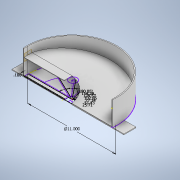
# Autodesk Inventor part: FlatRotationalTransferOldV
Saved by Autodesk Inventor 2020 (Build 240168000, 168)
## iProperties
Created: 2021-03-21
Part Number: FlatRotationalTransferOldV
Material: Generic
Document SubType Name: Sheet Metal
Designer: tdmp4
Density: 1 g/cm^3
Appearance: Default
Sheet Metal Rule: Default
Author: tdmp4
Autodesk Inventor part; units mm, degrees
ref_plane "YZ Plane" through (0, 0, 0) normal (1, 0, 0) x (0, 1, 0)
ref_plane "XZ Plane" through (0, 0, 0) normal (0, 1, 0) x (-1, 0, 0)
ref_plane "XY Plane" through (0, 0, 0) normal (0, 0, 1) x (1, 0, 0)
sketch "Sketch3" plane through (0, 0, 0) normal (0, 1, 0) x (-1, 0, 0)
  arc A0 (127.5964, -8.854) -> (151.8036, -8.854) centre (139.7, -12.7) ccw
  arc A1 (0, -12.7) -> (279.4, -12.7) centre (139.7, -12.7) ccw
  line L0 (279.4, -12.7) -> (279.4, 0)
  line L1 (279.4, 0) -> (151.8036, 0)
  line L2 (151.8036, 0) -> (151.8036, -8.854)
  line L3 (127.5964, 0) -> (0, 0)
  line L4 (0, 0) -> (0, -12.7)
  line L5 (127.5964, 0) -> (127.5964, -8.854)
  point P0 (0, -12.7)
  dimension "d9" = 279.4
  constraints: 12 end point, 4 point on circle, 3 vertical, 2 centre point, 2 perpendicular, 1 coincident, 1 point on line
  measures "d9" diameter of A1
extrude "Extrusion2" add sketch "Sketch3" along normal blind 2.54
sketch "Sketch4" plane through (0, 2.54, 0) normal (0, 1, 0) x (1, 0, 0)
  arc A0 (-127.5964, 8.854) -> (-151.8036, 8.854) centre (-139.7, 12.7) ccw projected
  arc A1 (0, 12.7) -> (-279.4, 12.7) centre (-139.7, 12.7) ccw
  line L0 (-127.5964, 0) -> (0, 0) projected
  line L1 (0, 0) -> (2.54, 0)
  line L2 (-279.4, 12.7) -> (-279.4, 0) projected
  line L3 (-279.4, 0) -> (-281.94, 0)
  circle A2 centre (-139.7, 12.7) radius 142.8058
  line L4 (0, 0) -> (2.54, 0)
  line L5 (0, 0) -> (0, 12.7)
  arc A3 (0, 12.7) -> (-279.4, 12.7) centre (-139.7, 12.7) ccw projected
  line L6 (-279.4, 0) -> (-279.4, 12.7)
  line L7 (-279.4, 0) -> (-281.94, 0)
  dimension "d12" = 2.54
  dimension "d13" = 2.54
  constraints: 13 end point, 3 point on circle, 2 coincident, 2 collinear, 2 point on line, 1 centre point, 1 horizontal, 1 perpendicular, 1 vertical, 3 other
  measures "d12" distance of L0.end L1.end
  measures "d13" distance of L2.end L3.end
extrude "Extrusion3" add sketch "Sketch4" along normal blind 76.2 contours A1 L2 L3 A2 L1 L5 picked at (-280.1039, 19.3593)
sketch "Sketch6" plane through (-279.4, 0, -12.7) normal (-1, 0, 0) x (0, 0, 1)
  line L0 (12.7, 0) -> (3.846, 0) projected
  line L1 (0, 2.54) -> (-139.7, 2.54) projected
  line L2 (12.7, 0) -> (-25.4, 0)
  line L3 (-25.4, 0) -> (-25.4, 2.54)
  line L4 (-25.4, 2.54) -> (12.7, 2.54)
  line L5 (12.7, 2.54) -> (12.7, 0)
  dimension "d16" = 38.1
  constraints: 8 end point, 2 parallel, 1 horizontal, 1 perpendicular, 1 point on line
  measures "d16" distance of L3.end L4.end
extrude "Extrusion4" add sketch "Sketch6" along normal mid plane 76.2
sketch "Sketch7" plane through (0, 0, 0) normal (1, 0, 0) x (0, 0, -1)
  line L0 (38.1, 0) -> (0, 0) projected
  line L1 (0, 0) -> (38.1, 0)
  line L2 (38.1, 0) -> (38.1, 2.54)
  line L3 (38.1, 2.54) -> (0, 2.54)
  line L4 (0, 2.54) -> (0, 0)
  dimension "d19" = 38.1
  dimension "d20" = 2.54
  constraints: 8 end point, 2 parallel, 1 horizontal, 1 perpendicular
  measures "d19" distance of L3.end L2.end
  measures "d20" distance of L1.end L2.end
extrude "Extrusion5" add sketch "Sketch7" along normal mid plane 76.2
sketch "Sketch8" plane through (0, 2.54, 0) normal (0, 1, 0) x (1, 0, 0)
  line L0 (-151.8036, 0) -> (-151.8036, 8.854) projected
  line L1 (-279.4, 0) -> (-151.8036, 0) projected
  line L2 (-151.8036, 0) -> (-279.4, 0)
  line L3 (-279.4, 0) -> (-279.4, 2.54)
  line L4 (-279.4, 12.7) -> (-279.4, 0) projected
  line L5 (-279.4, 2.54) -> (-151.8036, 2.54)
  line L6 (-151.8036, 2.54) -> (-151.8036, 0)
  arc A0 (-127.5964, 8.854) -> (-151.8036, 8.854) centre (-139.7, 12.7) ccw projected
  line L7 (-139.7, 12.7) -> (-15.4667, 72.5276)
  line L8 (-139.7, 12.7) -> (-1.8115, 12.7) construction
  line L9 (-139.7, 12.7) -> (-52.5985, 121.9219)
  arc A1 (-2.3285, 38.1) -> (-277.0715, 38.1) centre (-139.7, 12.7) ccw projected
  line L10 (-139.7, 12.7) -> (0, 12.7) construction
  line L11 (-139.7, 12.7) -> (-108.6138, 148.8974)
  line L12 (-139.7, 12.7) -> (0, 12.7) construction
  line L13 (-139.7, 12.7) -> (-170.7862, 148.8974)
  line L14 (-139.7, 12.7) -> (0, 12.7) construction
  line L15 (-139.7, 12.7) -> (-226.8015, 121.9219)
  line L16 (-139.7, 12.7) -> (0, 12.7) construction
  line L17 (-139.7, 12.7) -> (-265.5654, 73.3136)
  line L18 (-139.7, 12.7) -> (0, 12.7) construction
  line L19 (-139.7, 12.7) -> (-279.4, 12.7)
  line L20 (-139.7, 12.7) -> (0, 12.7) construction
  line L21 (-134.1897, 24.1423) -> (-105.865, 148.2407)
  line L22 (-127.3184, 15.526) -> (-11.7903, 68.8712)
  line L23 (-15.4667, 72.5276) -> (-11.0364, 74.6611)
  arc A2 (0.8288, 38.1) -> (-280.2288, 38.1) centre (-139.7, 12.7) ccw projected
  line L24 (-129.5192, 20.2922) -> (-47.6995, 121.9219)
  line L25 (-145.2103, 24.1423) -> (-173.535, 148.2407)
  line L26 (-149.8808, 20.2922) -> (-231.2375, 122.3102)
  line L27 (-152.0816, 15.526) -> (-266.5148, 71.3012)
  line L28 (-152.0816, 15.526) -> (-282.4779, 15.526)
  arc A3 (2.54, 0) -> (-281.94, 0) centre (-139.7, 12.7) ccw projected
  line L29 (-151.8036, 0) -> (-151.8036, 8.854)
  line L30 (-279.4, 0) -> (-151.8036, 0)
  line L31 (-151.8036, 0) -> (-279.4, 0)
  line L32 (-279.4, 0) -> (-279.4, 2.54)
  line L33 (-279.4, 12.7) -> (-279.4, 0)
  line L34 (-279.4, 2.54) -> (-151.8036, 2.54)
  line L35 (-151.8036, 2.54) -> (-151.8036, 0)
  arc A4 (-127.5964, 8.854) -> (-151.8036, 8.854) centre (-139.7, 12.7) ccw
  line L36 (-139.7, 12.7) -> (-15.4667, 72.5276)
  line L37 (-139.7, 12.7) -> (-1.8115, 12.7) construction
  line L38 (-139.7, 12.7) -> (-52.5985, 121.9219)
  arc A5 (-2.3285, 38.1) -> (-277.0715, 38.1) centre (-139.7, 12.7) ccw
  line L39 (-139.7, 12.7) -> (0, 12.7) construction
  line L40 (-139.7, 12.7) -> (-108.6138, 148.8974)
  line L41 (-139.7, 12.7) -> (0, 12.7) construction
  line L42 (-139.7, 12.7) -> (-170.7862, 148.8974)
  line L43 (-139.7, 12.7) -> (0, 12.7) construction
  line L44 (-139.7, 12.7) -> (-226.8015, 121.9219)
  line L45 (-139.7, 12.7) -> (0, 12.7) construction
  line L46 (-139.7, 12.7) -> (-265.5654, 73.3136)
  line L47 (-139.7, 12.7) -> (0, 12.7) construction
  line L48 (-139.7, 12.7) -> (-279.4, 12.7)
  line L49 (-139.7, 12.7) -> (0, 12.7) construction
  line L50 (-134.1897, 24.1423) -> (-105.865, 148.2407)
  line L51 (-127.3184, 15.526) -> (-11.7903, 68.8712)
  line L52 (-15.4667, 72.5276) -> (-11.0364, 74.6611)
  arc A6 (0.8288, 38.1) -> (-280.2288, 38.1) centre (-139.7, 12.7) ccw
  line L53 (-129.5192, 20.2922) -> (-47.6995, 121.9219)
  line L54 (-145.2103, 24.1423) -> (-173.535, 148.2407)
  line L55 (-149.8808, 20.2922) -> (-231.2375, 122.3102)
  line L56 (-152.0816, 15.526) -> (-266.5148, 71.3012)
  line L57 (-152.0816, 15.526) -> (-282.4779, 15.526)
  arc A7 (2.54, 0) -> (-281.94, 0) centre (-139.7, 12.7) ccw
  arc A8 (-277.0715, 38.1) -> (-279.4, 12.7) centre (-139.7, 12.7) ccw projected
  line L58 (-279.4, 12.7) -> (-279.3714, 15.526)
  point P0 (0, 0)
  point P1 (-13.8346, 73.3136)
  point P2 (-128.2577, 18.2103)
  point P3 (0, 0)
  point P4 (-13.8346, 73.3136)
  point P5 (-128.2577, 18.2103)
  point P6 (-49.6477, 119.502)
  point P7 (-131.7817, 22.6293)
  point P8 (-136.874, 25.0816)
  point P9 (-142.526, 25.0816)
  point P10 (-229.3005, 119.8813)
  point P11 (-147.6183, 22.6293)
  point P12 (-151.1423, 18.2103)
  dimension "d23" = 2.54
  dimension "d24" = 25.714
  dimension "d25" = 51.429
  dimension "d26" = 77.143
  dimension "d27" = 102.857
  dimension "d28" = 128.571
  dimension "d29" = 154.286
  dimension "d30" = 180
  dimension "d33" = 2.54
  dimension "d34" = 25.714
  dimension "d35" = 51.429
  dimension "d36" = 77.143
  dimension "d37" = 102.857
  dimension "d38" = 128.571
  dimension "d39" = 154.286
  dimension "d40" = 180
  constraints: 112 end point, 27 point on circle, 20 horizontal, 14 equal length, 4 parallel, 4 perpendicular, 3 centre point, 3 point on line, 23 other
  measures "d23" distance of L1.start L3.end
  measures "d24" angle of L8 L7
  measures "d25" angle of L10 L9
  measures "d26" angle of L12 L11
  measures "d27" angle of L14 L13
  measures "d28" angle of L16 L15
  measures "d29" angle of L18 L17
  measures "d30" angle of L19 L20
  measures "d33" distance of L30.start L32.end
  measures "d34" angle of L37 L36
  measures "d35" angle of L39 L38
  measures "d36" angle of L41 L40
  measures "d37" angle of L43 L42
  measures "d38" angle of L45 L44
  measures "d39" angle of L47 L46
  measures "d40" angle of L48 L49
sketch "Sketch10" plane through (0, 2.54, 0) normal (0, 1, 0) x (1, 0, 0)
  arc A0 (-36.5718, 0) -> (-230.6482, 12.6651) centre (-133.61, 6.3326) ccw
  line L0 (-127.5964, 8.854) -> (-127.5964, 0) projected
  point P0 (0, 0)
  constraints: 2 point on circle, 1 centre point
sketch "Sketch11" plane through (0, 2.54, 0) normal (0, 1, 0) x (1, 0, 0)
  line L0 (-127.5964, 8.854) -> (-127.5964, 0) projected
  line L1 (-127.5964, 0) -> (-151.8036, 0)
  line L2 (-139.7, 12.7038) -> (-139.7, 0)
  point P0 (0, 0)
  constraints: 4 end point, 1 horizontal, 1 midpoint
sketch "Sketch9" plane through (-127.5964, 2.54, 0) normal (0, 0, 1) x (1, 0, 0)
  line L0 (127.5964, 0) -> (127.5964, 76.2) projected
  line L1 (0, -2.54) -> (0, 0) projected
  line L2 (127.5964, 0) -> (0, 0)
  line L3 (0, 0) -> (0, 1.5578)
  line L4 (0, 1.5578) -> (127.5964, 1.5578)
  line L5 (127.5964, 1.5578) -> (127.5964, 0)
  point P0 (127.5964, -2.54)
  constraints: 8 end point, 4 perpendicular
sketch3d "3D Sketch3"
  helix H0 starts at (0, 2.54, -12.7) axis through (-139.7, 2.54, -12.7) along (0, 1, 0) pitch 101.6 turns 0.5 hand right
sweep "Sweep1" add profiles "Sketch9" path "3D Sketch3"
ref_plane "Work Plane1" through (-151.8036, 54.1189, -25.4) normal (0, 0, 1) x (1, 0, 0)
sketch "Sketch12" plane through (-151.8036, 54.1189, -25.4) normal (0, 0, 1) x (1, 0, 0)
  line L0 (0, 0.7789) -> (-127.0179, 0.7789) projected
  line L1 (0, -0.7789) -> (0, 0.7789) projected
  line L2 (-127.0179, 0.7789) -> (0, 0.7789)
  line L3 (0, 0.7789) -> (0, -0.7789)
  line L4 (0, -0.7789) -> (-127.0179, -0.7789)
  line L5 (-127.0179, -0.7789) -> (-127.0179, 0.7789)
  point P0 (151.8036, -54.1189)
  constraints: 8 end point, 2 parallel, 1 horizontal, 1 perpendicular
extrude "Extrusion13" add sketch "Sketch12" along normal blind 25.4
sketch "Sketch13" plane through (-278.8215, 54.8978, -25.4) normal (0, 1, 0) x (1, 0, 0)
  circle A0 centre (139.8334, -10.2382) radius 12.6074
  point P0 (278.8215, -25.4)
  constraints: 1 centre point
ref_plane "Work Plane2" through (-279.4, 53.34, -12.7) normal (1, 0, 0) x (0, 1, 0)
sketch "Sketch15" plane through (-279.4, 53.34, -12.7) normal (1, 0, 0) x (0, 1, 0)
  line L0 (-50.8, 0) -> (25.4, 0) projected
  circle A0 centre (-1.3792, 0) radius 1.3817
  point P0 (-53.34, 12.7)
  constraints: 1 centre point, 1 point on line
extrude "Extrusion15" cut sketch "Sketch15" along normal mid plane 20.6375
equation "\"BendRadius\" = Thickness"
equation "\"BendReliefWidth\" = Thickness"
equation "\"BendReliefDepth\" = 0.5 * Thickness"
equation "\"CornerReliefSize\" = 4 * Thickness"
equation "\"MinimumRemnant\" = 2 * Thickness"
equation "\"TransitionRadius\" = BendRadius"
equation "\"JacobiRadiusSize\" = Thickness"
equation "\"GapSize\" = Thickness"
equation "\"Thickness\" = 3.048"
body "Solid2"
